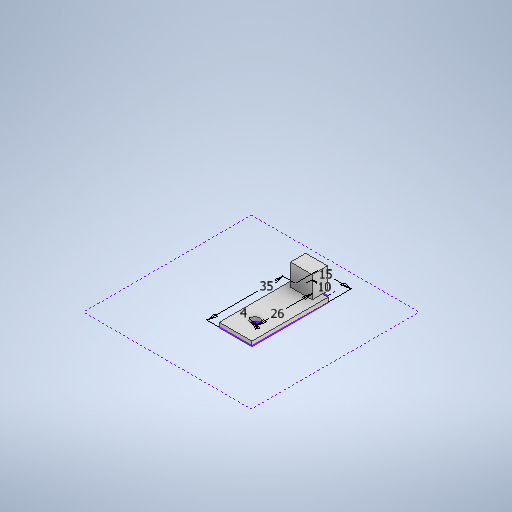
# Autodesk Inventor part: Sensor ky-037
Saved by Autodesk Inventor 2025.1 (Build 291241000, 241)
## iProperties
Created: 2025-03-25
Part Number: Sensor ky-037
Material: Generic
Document SubType Name: Modeling
Designer: maxwe
Density: 1 g/cm^3
Appearance: Default
Author: maxwe
Autodesk Inventor part; units mm, degrees
ref_plane "YZ Plane" through (0, 0, 0) normal (1, 0, 0) x (0, 1, 0)
ref_plane "XZ Plane" through (0, 0, 0) normal (0, 1, 0) x (-1, 0, 0)
ref_plane "XY Plane" through (0, 0, 0) normal (0, 0, 1) x (1, 0, 0)
sketch "Sketch1" plane through (0, 0, 0) normal (0, 1, 0) x (-1, 0, 0)
  line L0 (-30.5042, 34.8296) -> (46.7212, 34.8296) construction
  line L1 (46.7212, 34.8296) -> (46.7212, -42.3958) construction
  line L2 (46.7212, -42.3958) -> (-30.5042, -42.3958) construction
  line L3 (-30.5042, -42.3958) -> (-30.5042, 34.8296) construction
  line L4 (9.3977, 9.6123) -> (-5.6023, 9.6123)
  line L5 (-5.6023, 9.6123) -> (-5.6023, -25.3877)
  line L6 (-5.6023, -25.3877) -> (9.3977, -25.3877)
  line L7 (9.3977, -25.3877) -> (9.3977, 9.6123)
  circle A0 centre (1.9748, 0.6123) radius 2
  line L8 (7.0091, -20.7009) -> (-2.9909, -20.7009)
  line L9 (-2.9909, -20.7009) -> (-2.9909, -27.705)
  line L10 (-2.9909, -27.705) -> (7.0091, -27.705)
  line L11 (7.0091, -27.705) -> (7.0091, -20.7009)
  dimension "d6" = 35
  dimension "d9" = 15
  dimension "d11" = 4
  dimension "d21" = 26
  dimension "d26" = 10
  constraints: 16 end point, 4 parallel, 2 horizontal, 2 perpendicular, 1 centre point, 2 other
  measures "d6" distance of L6.end L4.start
  measures "d9" distance of L5.end L6.end
  measures "d11" diameter of A0
  measures "d21" distance from line of L6 A0.centre
  measures "d26" distance of L9.end L10.end
extrude "Extrusion1" add sketch "Sketch1" along normal blind 2 contours L7 L6 L11 L8 L9 L5 L4 | L6 L9 L8 L11
extrude "Extrusion2" add sketch "Sketch1" along normal blind 10 from surface at 2 contours L11 L10 L9 L6 | L6 L9 L8 L11
body "Solid1"
